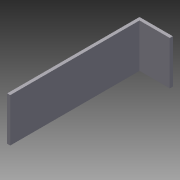
# Autodesk Inventor part: l_bracket
Saved by Autodesk Inventor 2011 (Build 150239000, 239)
## iProperties
Created: 2012-06-14
Part Number: l_bracket
Document SubType Name: Modeling
Designer: labuser
Density: 2.71 g/cm^3
Material: Aluminum-6061
Mass: 1809.8 g
Surface Area: 1525.76 cm^2
Volume: 667.824 cm^3
Author: labuser
Autodesk Inventor part; units mm, degrees
ref_plane "YZ Plane" through (0, 0, 0) normal (1, 0, 0) x (0, 1, 0)
ref_plane "XZ Plane" through (0, 0, 0) normal (0, 1, 0) x (-1, 0, 0)
ref_plane "XY Plane" through (0, 0, 0) normal (0, 0, 1) x (1, 0, 0)
sketch "Sketch1" plane through (0, 0, 0) normal (0, 0, 1) x (1, 0, 0)
  line L0 (0, 0) -> (104.775, 0)
  line L1 (104.775, 0) -> (104.775, 137.16)
  line L2 (104.775, 137.16) -> (0, 137.16)
  line L3 (0, 137.16) -> (0, 0)
  dimension "d0" = 104.775
  dimension "d1" = 137.16
  constraints: 8 end point, 2 parallel, 1 horizontal, 1 perpendicular
  measures "d0" distance of L2.end L1.end
  measures "d1" distance of L1.end L0.end
extrude "Extrusion1" add sketch "Sketch1" along normal blind 9.525
sketch "Sketch2" plane through (0, 0, 9.525) normal (0, 0, 1) x (1, 0, 0)
  line L0 (0, 137.16) -> (104.775, 137.16) projected
  line L1 (0, 0) -> (9.525, 0)
  line L2 (9.525, 0) -> (9.525, 137.16)
  line L3 (9.525, 137.16) -> (0, 137.16)
  line L4 (0, 137.16) -> (0, 0)
  dimension "d4" = 9.525
  constraints: 8 end point, 2 parallel, 1 horizontal, 1 perpendicular, 1 point on line
  measures "d4" distance of L3.end L2.end
extrude "Extrusion2" add sketch "Sketch2" along normal blind 406.4
body "Solid1"
